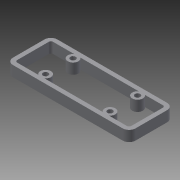
# Autodesk Inventor part: dualBaccable-ucan_fysect_middle
Saved by Autodesk Inventor 2014 SP2 (Build 180246200, 246)
## iProperties
Created: 2025-01-14
Part Number: dualBaccable-ucan_fysect_middle
Material: Generic
Document SubType Name: Sheet Metal
Designer: GauchoHP
Density: 1 g/cm^3
Sheet Metal Rule: Default_mm
Appearance: Default
Author: GauchoHP
Autodesk Inventor part; units mm, degrees
ref_plane "YZ Plane" through (0, 0, 0) normal (1, 0, 0) x (0, 1, 0)
ref_plane "XZ Plane" through (0, 0, 0) normal (0, 1, 0) x (-1, 0, 0)
ref_plane "XY Plane" through (0, 0, 0) normal (0, 0, 1) x (1, 0, 0)
sketch "Sketch1" plane through (0, 0, 0) normal (0, 0, 1) x (1, 0, 0)
  line L0 (-8.8921, 9.8249) -> (43.1079, 9.8249)
  line L1 (46.1079, 6.8249) -> (46.1079, -8.1751)
  line L2 (43.1079, -11.1751) -> (-8.8921, -11.1751)
  line L3 (-11.8921, -8.1751) -> (-11.8921, 6.8249)
  arc A0 (-8.8921, 9.8249) -> (-11.8921, 6.8249) centre (-8.8921, 6.8249) ccw
  arc A1 (46.1079, 6.8249) -> (43.1079, 9.8249) centre (43.1079, 6.8249) ccw
  arc A2 (43.1079, -11.1751) -> (46.1079, -8.1751) centre (43.1079, -8.1751) ccw
  arc A3 (-11.8921, -8.1751) -> (-8.8921, -11.1751) centre (-8.8921, -8.1751) ccw
  line L4 (43.1079, 7.8249) -> (-8.8921, 7.8249)
  arc A4 (-8.8921, 7.8249) -> (-9.8921, 6.8249) centre (-8.8921, 6.8249) ccw
  line L5 (-9.8921, 6.8249) -> (-9.8921, -8.1751)
  arc A5 (-9.8921, -8.1751) -> (-8.8921, -9.1751) centre (-8.8921, -8.1751) ccw
  line L6 (-8.8921, -9.1751) -> (43.1079, -9.1751)
  arc A6 (43.1079, -9.1751) -> (44.1079, -8.1751) centre (43.1079, -8.1751) ccw
  line L7 (44.1079, -8.1751) -> (44.1079, 6.8249)
  arc A7 (44.1079, 6.8249) -> (43.1079, 7.8249) centre (43.1079, 6.8249) ccw
  circle A8 centre (2.6079, -7.1751) radius 2.5
  circle A9 centre (2.6079, -7.1751) radius 1.25
  circle A10 centre (2.6079, 5.8249) radius 2.5
  circle A11 centre (2.6079, 5.8249) radius 1.25
  circle A12 centre (33.1079, 5.8249) radius 2.5
  circle A13 centre (33.1079, 5.8249) radius 1.25
  circle A14 centre (33.1079, -7.1751) radius 2.5
  circle A15 centre (33.1079, -7.1751) radius 1.25
  point P0 (0, 0)
  point P1 (-11.8921, 9.8249)
  point P2 (46.1079, 9.8249)
  point P3 (-11.8921, -11.1751)
  dimension "d0" = 58
  dimension "d1" = 21
  dimension "d2" = 3
  dimension "d5" = 2
  dimension "d6" = 5
  dimension "d7" = 2.5
  dimension "d8" = 5
  dimension "d9" = 2.5
  dimension "d10" = 5
  dimension "d11" = 2.5
  dimension "d12" = 5
  dimension "d13" = 2.5
  dimension "d14" = 30.5
  dimension "d15" = 30.5
  dimension "d16" = 13
  dimension "d17" = 2
  dimension "d18" = 11
  dimension "d19" = 11
  constraints: 16 centre point, 16 end point, 16 point on circle, 8 tangent, 6 point on line, 4 coincident, 4 parallel, 3 equal radius, 2 perpendicular, 1 horizontal, 7 other
  measures "d0" distance of point (-11.892, 9.825) point (46.108, 9.825)
  measures "d1" distance of point (-11.892, -11.175) point (-11.892, 9.825)
  measures "d2" radius of A0
  measures "d5" distance between parallel lines of L4 L0
  measures "d6" diameter of A8
  measures "d7" diameter of A9
  measures "d8" diameter of A10
  measures "d9" diameter of A11
  measures "d10" diameter of A12
  measures "d11" diameter of A13
  measures "d12" diameter of A14
  measures "d13" diameter of A15
  measures "d14" distance of A12.centre A10.centre
  measures "d15" distance of A14.centre A8.centre
  measures "d16" distance of A8.centre A10.centre
  measures "d17" distance from line of L6 A8.centre
  measures "d18" distance from line of L7 A12.centre
  measures "d19" distance from line of L7 A14.centre
extrude "Extrusion1" add sketch "Sketch1" along normal blind 5 contours L0 A1 L1 A2 L2 A3 L3 A0 | A12 L4 | L4 A12 | A10 L4 | L4 A10 | A14 L6 | L6 A14 | A8 L6 | L6 A8
equation "\"BendRadius\" = Thickness"
equation "\"BendReliefWidth\" = Thickness"
equation "\"BendReliefDepth\" = 0.5 * Thickness"
equation "\"CornerReliefSize\" = 4 * Thickness"
equation "\"MinimumRemnant\" = 2 * Thickness"
equation "\"TransitionRadius\" = BendRadius"
equation "\"JacobiRadiusSize\" = BendRadius"
equation "\"GapSize\" = Thickness"
equation "\"Thickness\" = 0.5"
body "Solid1"
